Autodesk Fusion 360 part; units mm, degrees
note: some values were not read from the file. Set by a fixed rule: which face or edge a step refers to.
(part 2 of 3)
sketch "Skizze9" plane through (0, 0, 0) normal (0, 0, -1) x (1, 0, 0)
  circle A0 centre (287.3074, 352.379) radius 12
  line L0 (376.8151, 422.379) -> (364.2997, 422.379)
  arc A1 (343.5151, 422.379) -> (364.2997, 422.379) centre (353.9074, 428.379) ccw
  line L1 (343.5151, 422.379) -> (330.9997, 422.379)
  arc A2 (310.2151, 422.379) -> (330.9997, 422.379) centre (320.6074, 428.379) ccw
  line L2 (310.2151, 422.379) -> (297.6997, 422.379)
  arc A3 (276.9151, 422.379) -> (297.6997, 422.379) centre (287.3074, 428.379) ccw
  line L3 (276.9151, 422.379) -> (264.3997, 422.379)
  arc A4 (243.6151, 422.379) -> (264.3997, 422.379) centre (254.0074, 428.379) ccw
  line L4 (243.6151, 422.379) -> (231.0997, 422.379)
  arc A5 (210.3151, 422.379) -> (231.0997, 422.379) centre (220.7074, 428.379) ccw
  line L5 (210.3151, 422.379) -> (197.7997, 422.379)
  arc A6 (177.0151, 422.379) -> (197.7997, 422.379) centre (187.4074, 428.379) ccw
  line L6 (177.0151, 422.379) -> (164.4997, 422.379)
  arc A7 (143.7151, 422.379) -> (164.4997, 422.379) centre (154.1074, 428.379) ccw
  line L7 (143.7151, 422.379) -> (131.1997, 422.379)
  arc A8 (110.4151, 422.379) -> (131.1997, 422.379) centre (120.8074, 428.379) ccw
  line L8 (110.4151, 422.379) -> (97.8997, 422.379)
  arc A9 (77.1151, 422.379) -> (97.8997, 422.379) centre (87.5074, 428.379) ccw
  line L9 (77.1151, 422.379) -> (60.1074, 422.379)
  line L10 (60.1074, 422.379) -> (60.1074, 64.779)
  line L11 (60.1074, 64.779) -> (447.9074, 64.779)
  line L12 (447.9074, 64.779) -> (447.9074, 422.379)
  line L13 (447.9074, 422.379) -> (430.8997, 422.379)
  arc A10 (410.1151, 422.379) -> (430.8997, 422.379) centre (420.5074, 428.379) ccw
  line L14 (410.1151, 422.379) -> (397.5997, 422.379)
  arc A11 (376.8151, 422.379) -> (397.5997, 422.379) centre (387.2074, 428.379) ccw
  circle A12 centre (420.5074, 390.379) radius 12
  circle A13 centre (387.2074, 390.379) radius 12
  circle A14 centre (353.9074, 390.379) radius 12
  circle A15 centre (320.6074, 390.379) radius 12
  circle A16 centre (287.3074, 390.379) radius 12
  circle A17 centre (254.0074, 390.379) radius 12
  circle A18 centre (220.7074, 390.379) radius 12
  circle A19 centre (187.4074, 390.379) radius 12
  circle A20 centre (154.1074, 390.379) radius 12
  circle A21 centre (120.8074, 390.379) radius 12
  circle A22 centre (87.5074, 390.379) radius 12
  circle A23 centre (420.5074, 352.379) radius 12
  circle A24 centre (387.2074, 352.379) radius 12
  circle A25 centre (353.9074, 352.379) radius 12
  circle A26 centre (320.6074, 352.379) radius 12
  circle A27 centre (420.5074, 124.379) radius 12
  circle A28 centre (87.5074, 162.379) radius 12
  circle A29 centre (120.8074, 162.379) radius 12
  circle A30 centre (154.1074, 162.379) radius 12
  circle A31 centre (187.4074, 162.379) radius 12
  circle A32 centre (220.7074, 162.379) radius 12
  circle A33 centre (254.0074, 162.379) radius 12
  circle A34 centre (287.3074, 162.379) radius 12
  circle A35 centre (320.6074, 162.379) radius 12
  circle A36 centre (353.9074, 162.379) radius 12
  circle A37 centre (387.2074, 162.379) radius 12
  circle A38 centre (420.5074, 162.379) radius 12
  circle A39 centre (87.5074, 200.379) radius 12
  circle A40 centre (120.8074, 200.379) radius 12
  circle A41 centre (154.1074, 200.379) radius 12
  circle A42 centre (187.4074, 200.379) radius 12
  circle A43 centre (220.7074, 200.379) radius 12
  circle A44 centre (254.0074, 200.379) radius 12
  circle A45 centre (287.3074, 200.379) radius 12
  circle A46 centre (320.6074, 200.379) radius 12
  circle A47 centre (353.9074, 200.379) radius 12
  circle A48 centre (387.2074, 200.379) radius 12
  circle A49 centre (420.5074, 200.379) radius 12
  circle A50 centre (87.5074, 238.379) radius 12
  circle A51 centre (120.8074, 238.379) radius 12
  circle A52 centre (154.1074, 238.379) radius 12
  circle A53 centre (187.4074, 238.379) radius 12
  circle A54 centre (220.7074, 238.379) radius 12
  circle A55 centre (254.0074, 238.379) radius 12
  circle A56 centre (287.3074, 238.379) radius 12
  circle A57 centre (320.6074, 238.379) radius 12
  circle A58 centre (353.9074, 238.379) radius 12
  circle A59 centre (254.0074, 352.379) radius 12
  circle A60 centre (220.7074, 352.379) radius 12
  circle A61 centre (187.4074, 352.379) radius 12
  circle A62 centre (154.1074, 352.379) radius 12
  circle A63 centre (120.8074, 352.379) radius 12
  circle A64 centre (87.5074, 352.379) radius 12
  circle A65 centre (420.5074, 314.379) radius 12
  circle A66 centre (387.2074, 314.379) radius 12
  circle A67 centre (353.9074, 314.379) radius 12
  circle A68 centre (320.6074, 314.379) radius 12
  circle A69 centre (287.3074, 314.379) radius 12
  circle A70 centre (254.0074, 314.379) radius 12
  circle A71 centre (220.7074, 314.379) radius 12
  circle A72 centre (187.4074, 314.379) radius 12
  circle A73 centre (154.1074, 314.379) radius 12
  circle A74 centre (120.8074, 314.379) radius 12
  circle A75 centre (87.5074, 314.379) radius 12
  circle A76 centre (420.5074, 276.379) radius 12
  circle A77 centre (387.2074, 276.379) radius 12
  circle A78 centre (353.9074, 276.379) radius 12
  circle A79 centre (320.6074, 276.379) radius 12
  circle A80 centre (287.3074, 276.379) radius 12
  circle A81 centre (254.0074, 276.379) radius 12
  circle A82 centre (220.7074, 276.379) radius 12
  circle A83 centre (187.4074, 276.379) radius 12
  circle A84 centre (154.1074, 276.379) radius 12
  circle A85 centre (120.8074, 276.379) radius 12
  circle A86 centre (87.5074, 276.379) radius 12
  circle A87 centre (420.5074, 238.379) radius 12
  circle A88 centre (387.2074, 238.379) radius 12
  circle A89 centre (87.5074, 86.379) radius 12
  circle A90 centre (120.8074, 86.379) radius 12
  circle A91 centre (154.1074, 86.379) radius 12
  circle A92 centre (187.4074, 86.379) radius 12
  circle A93 centre (220.7074, 86.379) radius 12
  circle A94 centre (254.0074, 86.379) radius 12
  circle A95 centre (287.3074, 86.379) radius 12
  circle A96 centre (320.6074, 86.379) radius 12
  circle A97 centre (353.9074, 86.379) radius 12
  circle A98 centre (387.2074, 86.379) radius 12
  circle A99 centre (420.5074, 86.379) radius 12
  circle A100 centre (87.5074, 124.379) radius 12
  circle A101 centre (120.8074, 124.379) radius 12
  circle A102 centre (154.1074, 124.379) radius 12
  circle A103 centre (187.4074, 124.379) radius 12
  circle A104 centre (220.7074, 124.379) radius 12
  circle A105 centre (254.0074, 124.379) radius 12
  circle A106 centre (287.3074, 124.379) radius 12
  circle A107 centre (320.6074, 124.379) radius 12
  circle A108 centre (353.9074, 124.379) radius 12
  circle A109 centre (387.2074, 124.379) radius 12
  line L15 (60.1074, 396.379) -> (447.9074, 396.379)
  line L16 (447.9074, 396.379) -> (447.9074, 384.379)
  line L17 (447.9074, 384.379) -> (60.1074, 384.379)
  line L18 (60.1074, 384.379) -> (60.1074, 396.379)
  dimension "d208" = 6
  dimension "d209" = 6
  constraint horizontal L15
  constraint vertical L16
  constraint horizontal L17
  constraint vertical L18
  constraint collinear L10 L18
  constraint collinear L12 L16
  measures "d208" distance of A22.centre L15
  measures "d209" distance of A22.centre L17
extrude "Extrusion8" cut sketch "Skizze9" against normal blind 1 contours L12 A12 L15 L16 L17 | A12 A13 L15 L17 | L10 A22 L15 L17 L18 | A13 A14 L15 L17 | A21 A22 L15 L17 | A14 A15 L15 L17 | A20 A21 L15 L17 | A15 A16 L15 L17 | A19 A20 L15 L17 | A16 A17 L15 L17 | A18 A19 L15 L17 | A17 A18 L15 L17
extrude "Extrusion9" cut 1 faces at (441.9014, -440.073, 0) along direction (0, 0, 1) blind 10
extrude "Extrusion10" cut 1 faces at (441.4947, -412.7802, 0) along direction (0, 0, 1) blind 10
extrude "Extrusion11" cut 1 faces at (442.774, -216.5124, 0) along direction (0, 0, 1) blind 10
extrude "Extrusion12" cut 24 faces at (338.8297, -428.379, 1) (205.6297, -428.379, 1) (372.1297, -428.379, 1) (65.2519, -428.6779, 1) (305.5297, -428.379, 1) (272.2297, -428.379, 1) (238.9297, -428.379, 1) (105.7297, -428.379, 1) (172.3297, -428.379, 1) (139.0297, -428.379, 1) (405.4297, -428.379, 1) (442.774, -428.379, 1) (65.2519, -390.0801, 1) (105.7297, -390.379, 1) (139.0297, -390.379, 1) (172.3297, -390.379, 1) (205.6297, -390.379, 1) (238.9297, -390.379, 1) (272.2297, -390.379, 1) (305.5297, -390.379, 1) (338.8297, -390.379, 1) (372.1297, -390.379, 1) (405.4297, -390.379, 1) (442.774, -390.379, 1) along direction (0, 0, 1) blind 10
sketch "Skizze10" plane through (0, 0, 0) normal (0, 0, -1) x (1, 0, 0)
  line L0 (50.1074, 9.779) -> (50.1074, 49.779)
  line L1 (50.1074, 49.779) -> (10.1074, 49.779)
  line L2 (10.1074, 49.779) -> (10.1074, 464.979)
  line L3 (10.1074, 464.979) -> (50.1074, 464.979)
  line L4 (50.1074, 464.979) -> (50.1074, 504.979)
  line L5 (50.1074, 504.979) -> (457.9074, 504.979)
  line L6 (457.9074, 504.979) -> (457.9074, 464.979)
  line L7 (457.9074, 464.979) -> (497.9074, 464.979)
  line L8 (497.9074, 464.979) -> (497.9074, 49.779)
  line L9 (497.9074, 49.779) -> (457.9074, 49.779)
  line L10 (457.9074, 49.779) -> (457.9074, 9.779)
  line L11 (457.9074, 9.779) -> (50.1074, 9.779)
  circle A0 centre (479.9074, 23.779) radius 12
  circle A1 centre (28.1074, 23.779) radius 10.8095
  circle A2 centre (28.1074, 490.979) radius 12
  circle A3 centre (479.9074, 490.979) radius 12
  line L12 (507.9074, 514.979) -> (0.1074, 514.979)
  line L13 (0.1074, 514.979) -> (0.1074, -0.221)
  line L14 (0.1074, -0.221) -> (507.9074, -0.221)
  line L15 (507.9074, -0.221) -> (507.9074, 514.979)
  line L16 (457.9074, 496.979) -> (497.9074, 496.979)
  line L17 (497.9074, 496.979) -> (497.9074, 484.979)
  line L18 (497.9074, 484.979) -> (457.9074, 484.979)
  line L19 (457.9074, 484.979) -> (457.9074, 496.979)
  dimension "d220" = 6
  dimension "d221" = 6
  constraint horizontal L16
  constraint vertical L17
  constraint horizontal L18
  constraint vertical L19
  constraint coincident L6 L16.start
  constraint collinear L8 L17
  measures "d220" distance of A3.centre L16
  measures "d221" distance of A3.centre L18
extrude "Extrusion13" cut sketch "Skizze10" against normal blind 5 contours L6 A3 L16 L18 L19 | A3 L16 L17 L18
sketch "Skizze11" plane through (0, 0, 0) normal (0, 0, -1) x (1, 0, 0)
  line L0 (507.9074, 514.979) -> (0.1074, 514.979)
  line L1 (0.1074, 514.979) -> (0.1074, -0.221)
  line L2 (0.1074, -0.221) -> (507.9074, -0.221)
  line L3 (507.9074, -0.221) -> (507.9074, 514.979)
  circle A0 centre (28.1074, 490.979) radius 12
  circle A1 centre (28.1074, 23.779) radius 10.8095
  circle A2 centre (479.9074, 23.779) radius 12
  line L4 (469.5151, 484.979) -> (457.9074, 484.979)
  line L5 (457.9074, 484.979) -> (457.9074, 464.979)
  line L6 (457.9074, 464.979) -> (497.9074, 464.979)
  line L7 (497.9074, 464.979) -> (497.9074, 49.779)
  line L8 (497.9074, 49.779) -> (457.9074, 49.779)
  line L9 (457.9074, 49.779) -> (457.9074, 9.779)
  line L10 (457.9074, 9.779) -> (50.1074, 9.779)
  line L11 (50.1074, 9.779) -> (50.1074, 49.779)
  line L12 (50.1074, 49.779) -> (10.1074, 49.779)
  line L13 (10.1074, 49.779) -> (10.1074, 464.979)
  line L14 (10.1074, 464.979) -> (50.1074, 464.979)
  line L15 (50.1074, 464.979) -> (50.1074, 504.979)
  line L16 (50.1074, 504.979) -> (457.9074, 504.979)
  line L17 (457.9074, 504.979) -> (457.9074, 496.979)
  line L18 (457.9074, 496.979) -> (469.5151, 496.979)
  arc A3 (490.2997, 496.979) -> (469.5151, 496.979) centre (479.9074, 490.979) ccw
  line L19 (490.2997, 496.979) -> (497.9074, 496.979)
  line L20 (497.9074, 496.979) -> (497.9074, 484.979)
  line L21 (497.9074, 484.979) -> (490.2997, 484.979)
  arc A4 (469.5151, 484.979) -> (490.2997, 484.979) centre (479.9074, 490.979) ccw
  line L22 (10.1074, 496.979) -> (50.1074, 496.979)
  line L23 (50.1074, 496.979) -> (50.1074, 484.979)
  line L24 (50.1074, 484.979) -> (10.1074, 484.979)
  line L25 (10.1074, 484.979) -> (10.1074, 496.979)
  dimension "d224" = 6
  dimension "d225" = 6
  constraint horizontal L22
  constraint vertical L23
  constraint horizontal L24
  constraint vertical L25
  constraint collinear L15 L23
  constraint collinear L13 L25
  measures "d224" distance of A0.centre L22
  measures "d225" distance of A0.centre L24
extrude "Extrusion14" cut sketch "Skizze11" against normal blind 6 contours A0 L15 L22 L23 L24 | A0 L22 L24 L25
sketch "Skizze12" plane through (0, 0, 0) normal (0, 0, -1) x (1, 0, 0)
  line L0 (50.1074, 484.979) -> (38.4997, 484.979)
  arc A0 (17.7151, 484.979) -> (38.4997, 484.979) centre (28.1074, 490.979) ccw
  line L1 (17.7151, 484.979) -> (10.1074, 484.979)
  line L2 (10.1074, 484.979) -> (10.1074, 496.979)
  line L3 (10.1074, 496.979) -> (17.7151, 496.979)
  arc A1 (38.4997, 496.979) -> (17.7151, 496.979) centre (28.1074, 490.979) ccw
  line L4 (38.4997, 496.979) -> (50.1074, 496.979)
  line L5 (50.1074, 496.979) -> (50.1074, 504.979)
  line L6 (50.1074, 504.979) -> (457.9074, 504.979)
  line L7 (457.9074, 504.979) -> (457.9074, 496.979)
  line L8 (457.9074, 496.979) -> (469.5151, 496.979)
  arc A2 (490.2997, 496.979) -> (469.5151, 496.979) centre (479.9074, 490.979) ccw
  line L9 (490.2997, 496.979) -> (497.9074, 496.979)
  line L10 (497.9074, 496.979) -> (497.9074, 484.979)
  line L11 (497.9074, 484.979) -> (490.2997, 484.979)
  arc A3 (469.5151, 484.979) -> (490.2997, 484.979) centre (479.9074, 490.979) ccw
  line L12 (469.5151, 484.979) -> (457.9074, 484.979)
  line L13 (457.9074, 484.979) -> (457.9074, 464.979)
  line L14 (457.9074, 464.979) -> (497.9074, 464.979)
  line L15 (497.9074, 464.979) -> (497.9074, 49.779)
  line L16 (497.9074, 49.779) -> (457.9074, 49.779)
  line L17 (457.9074, 49.779) -> (457.9074, 9.779)
  line L18 (457.9074, 9.779) -> (50.1074, 9.779)
  line L19 (50.1074, 9.779) -> (50.1074, 49.779)
  line L20 (50.1074, 49.779) -> (10.1074, 49.779)
  line L21 (10.1074, 49.779) -> (10.1074, 464.979)
  line L22 (10.1074, 464.979) -> (50.1074, 464.979)
  line L23 (50.1074, 464.979) -> (50.1074, 484.979)
  line L24 (507.9074, 514.979) -> (0.1074, 514.979)
  line L25 (0.1074, 514.979) -> (0.1074, -0.221)
  line L26 (0.1074, -0.221) -> (507.9074, -0.221)
  line L27 (507.9074, -0.221) -> (507.9074, 514.979)
  circle A4 centre (28.1074, 23.779) radius 10.8095
  circle A5 centre (479.9074, 23.779) radius 12
  line L28 (10.1074, 29.779) -> (50.1074, 29.779)
  line L29 (50.1074, 29.779) -> (50.1074, 17.779)
  line L30 (50.1074, 17.779) -> (10.1074, 17.779)
  line L31 (10.1074, 17.779) -> (10.1074, 29.779)
  dimension "d228" = 6
  dimension "d229" = 6
  constraint horizontal L28
  constraint vertical L29
  constraint horizontal L30
  constraint vertical L31
  constraint collinear L19 L29
  constraint collinear L21 L31
  measures "d228" distance of A4.centre L28
  measures "d229" distance of A4.centre L30
extrude "Extrusion15" cut sketch "Skizze12" against normal blind 6 contours L19 A4 L28 L29 L30 | A4 L28 L30 L31
sketch "Skizze13" plane through (0, 0, 0) normal (0, 0, -1) x (1, 0, 0)
  line L0 (50.1074, 17.779) -> (37.0987, 17.779)
  arc A0 (19.116, 17.779) -> (37.0987, 17.779) centre (28.1074, 23.779) ccw
  line L1 (19.116, 17.779) -> (10.1074, 17.779)
  line L2 (10.1074, 17.779) -> (10.1074, 29.779)
  line L3 (10.1074, 29.779) -> (19.116, 29.779)
  arc A1 (37.0987, 29.779) -> (19.116, 29.779) centre (28.1074, 23.779) ccw
  line L4 (37.0987, 29.779) -> (50.1074, 29.779)
  line L5 (50.1074, 29.779) -> (50.1074, 49.779)
  line L6 (50.1074, 49.779) -> (10.1074, 49.779)
  line L7 (10.1074, 49.779) -> (10.1074, 464.979)
  line L8 (10.1074, 464.979) -> (50.1074, 464.979)
  line L9 (50.1074, 464.979) -> (50.1074, 484.979)
  line L10 (50.1074, 484.979) -> (38.4997, 484.979)
  arc A2 (17.7151, 484.979) -> (38.4997, 484.979) centre (28.1074, 490.979) ccw
  line L11 (17.7151, 484.979) -> (10.1074, 484.979)
  line L12 (10.1074, 484.979) -> (10.1074, 496.979)
  line L13 (10.1074, 496.979) -> (17.7151, 496.979)
  arc A3 (38.4997, 496.979) -> (17.7151, 496.979) centre (28.1074, 490.979) ccw
  line L14 (38.4997, 496.979) -> (50.1074, 496.979)
  line L15 (50.1074, 496.979) -> (50.1074, 504.979)
  line L16 (50.1074, 504.979) -> (457.9074, 504.979)
  line L17 (457.9074, 504.979) -> (457.9074, 496.979)
  line L18 (457.9074, 496.979) -> (469.5151, 496.979)
  arc A4 (490.2997, 496.979) -> (469.5151, 496.979) centre (479.9074, 490.979) ccw
  line L19 (490.2997, 496.979) -> (497.9074, 496.979)
  line L20 (497.9074, 496.979) -> (497.9074, 484.979)
  line L21 (497.9074, 484.979) -> (490.2997, 484.979)
  arc A5 (469.5151, 484.979) -> (490.2997, 484.979) centre (479.9074, 490.979) ccw
  line L22 (469.5151, 484.979) -> (457.9074, 484.979)
  line L23 (457.9074, 484.979) -> (457.9074, 464.979)
  line L24 (457.9074, 464.979) -> (497.9074, 464.979)
  line L25 (497.9074, 464.979) -> (497.9074, 49.779)
  line L26 (497.9074, 49.779) -> (457.9074, 49.779)
  line L27 (457.9074, 49.779) -> (457.9074, 9.779)
  line L28 (457.9074, 9.779) -> (50.1074, 9.779)
  line L29 (50.1074, 9.779) -> (50.1074, 17.779)
  line L30 (507.9074, 514.979) -> (0.1074, 514.979)
  line L31 (0.1074, 514.979) -> (0.1074, -0.221)
  line L32 (0.1074, -0.221) -> (507.9074, -0.221)
  line L33 (507.9074, -0.221) -> (507.9074, 514.979)
  circle A6 centre (479.9074, 23.779) radius 12
  line L34 (457.9074, 29.779) -> (497.9074, 29.779)
  line L35 (497.9074, 29.779) -> (497.9074, 17.779)
  line L36 (497.9074, 17.779) -> (457.9074, 17.779)
  line L37 (457.9074, 17.779) -> (457.9074, 29.779)
  dimension "d232" = 6
  dimension "d233" = 6
  constraint horizontal L34
  constraint vertical L35
  constraint horizontal L36
  constraint vertical L37
  constraint collinear L25 L35
  constraint collinear L27 L37
  measures "d232" distance of A6.centre L34
  measures "d233" distance of A6.centre L36
extrude "Extrusion16" cut sketch "Skizze13" against normal blind 6 contours L27 A6 L34 L36 L37 | A6 L34 L35 L36
sketch "Skizze14" plane through (0, 0, 10) normal (0, 0, -1) x (1, 0, 0)
  circle A0 centre (387.2074, 124.379) radius 12
  circle A1 centre (353.9074, 124.379) radius 12
  circle A2 centre (320.6074, 124.379) radius 12
  circle A3 centre (287.3074, 124.379) radius 12
  circle A4 centre (254.0074, 124.379) radius 12
  circle A5 centre (220.7074, 124.379) radius 12
  circle A6 centre (187.4074, 124.379) radius 12
  circle A7 centre (154.1074, 124.379) radius 12
  circle A8 centre (120.8074, 124.379) radius 12
  circle A9 centre (87.5074, 124.379) radius 12
  circle A10 centre (420.5074, 86.379) radius 12
  circle A11 centre (387.2074, 86.379) radius 12
  circle A12 centre (353.9074, 86.379) radius 12
  circle A13 centre (320.6074, 86.379) radius 12
  circle A14 centre (287.3074, 86.379) radius 12
  circle A15 centre (254.0074, 86.379) radius 12
  circle A16 centre (220.7074, 86.379) radius 12
  circle A17 centre (187.4074, 86.379) radius 12
  circle A18 centre (154.1074, 86.379) radius 12
  circle A19 centre (120.8074, 86.379) radius 12
  circle A20 centre (87.5074, 86.379) radius 12
  circle A21 centre (387.2074, 238.379) radius 12
  circle A22 centre (420.5074, 238.379) radius 12
  circle A23 centre (87.5074, 276.379) radius 12
  circle A24 centre (120.8074, 276.379) radius 12
  circle A25 centre (154.1074, 276.379) radius 12
  circle A26 centre (187.4074, 276.379) radius 12
  circle A27 centre (220.7074, 276.379) radius 12
  circle A28 centre (254.0074, 276.379) radius 12
  circle A29 centre (287.3074, 276.379) radius 12
  circle A30 centre (320.6074, 276.379) radius 12
  circle A31 centre (353.9074, 276.379) radius 12
  circle A32 centre (387.2074, 276.379) radius 12
  circle A33 centre (420.5074, 276.379) radius 12
  circle A34 centre (87.5074, 314.379) radius 12
  circle A35 centre (120.8074, 314.379) radius 12
  circle A36 centre (154.1074, 314.379) radius 12
  circle A37 centre (187.4074, 314.379) radius 12
  circle A38 centre (220.7074, 314.379) radius 12
  circle A39 centre (254.0074, 314.379) radius 12
  circle A40 centre (287.3074, 314.379) radius 12
  circle A41 centre (320.6074, 314.379) radius 12
  circle A42 centre (353.9074, 314.379) radius 12
  circle A43 centre (387.2074, 314.379) radius 12
  circle A44 centre (420.5074, 314.379) radius 12
  circle A45 centre (87.5074, 352.379) radius 12
  circle A46 centre (120.8074, 352.379) radius 12
  circle A47 centre (154.1074, 352.379) radius 12
  circle A48 centre (187.4074, 352.379) radius 12
  circle A49 centre (220.7074, 352.379) radius 12
  circle A50 centre (254.0074, 352.379) radius 12
  circle A51 centre (353.9074, 238.379) radius 12
  circle A52 centre (320.6074, 238.379) radius 12
  circle A53 centre (287.3074, 238.379) radius 12
  circle A54 centre (254.0074, 238.379) radius 12
  circle A55 centre (220.7074, 238.379) radius 12
  circle A56 centre (187.4074, 238.379) radius 12
  circle A57 centre (154.1074, 238.379) radius 12
  circle A58 centre (120.8074, 238.379) radius 12
  circle A59 centre (87.5074, 238.379) radius 12
  circle A60 centre (420.5074, 200.379) radius 12
  circle A61 centre (387.2074, 200.379) radius 12
  circle A62 centre (353.9074, 200.379) radius 12
  circle A63 centre (320.6074, 200.379) radius 12
  circle A64 centre (287.3074, 200.379) radius 12
  circle A65 centre (254.0074, 200.379) radius 12
  circle A66 centre (220.7074, 200.379) radius 12
  circle A67 centre (187.4074, 200.379) radius 12
  circle A68 centre (154.1074, 200.379) radius 12
  circle A69 centre (120.8074, 200.379) radius 12
  circle A70 centre (87.5074, 200.379) radius 12
  circle A71 centre (420.5074, 162.379) radius 12
  circle A72 centre (387.2074, 162.379) radius 12
  circle A73 centre (353.9074, 162.379) radius 12
  circle A74 centre (320.6074, 162.379) radius 12
  circle A75 centre (287.3074, 162.379) radius 12
  circle A76 centre (254.0074, 162.379) radius 12
  circle A77 centre (220.7074, 162.379) radius 12
  circle A78 centre (187.4074, 162.379) radius 12
  circle A79 centre (154.1074, 162.379) radius 12
  circle A80 centre (120.8074, 162.379) radius 12
  circle A81 centre (87.5074, 162.379) radius 12
  circle A82 centre (420.5074, 124.379) radius 12
  circle A83 centre (320.6074, 352.379) radius 12
  circle A84 centre (353.9074, 352.379) radius 12
  circle A85 centre (387.2074, 352.379) radius 12
  circle A86 centre (420.5074, 352.379) radius 12
  line L0 (376.8151, 384.379) -> (364.2997, 384.379)
  arc A87 (343.5151, 384.379) -> (364.2997, 384.379) centre (353.9074, 390.379) ccw
  line L1 (343.5151, 384.379) -> (330.9997, 384.379)
  arc A88 (310.2151, 384.379) -> (330.9997, 384.379) centre (320.6074, 390.379) ccw
  line L2 (310.2151, 384.379) -> (297.6997, 384.379)
  arc A89 (276.9151, 384.379) -> (297.6997, 384.379) centre (287.3074, 390.379) ccw
  line L3 (276.9151, 384.379) -> (264.3997, 384.379)
  arc A90 (243.6151, 384.379) -> (264.3997, 384.379) centre (254.0074, 390.379) ccw
  line L4 (243.6151, 384.379) -> (231.0997, 384.379)
  arc A91 (210.3151, 384.379) -> (231.0997, 384.379) centre (220.7074, 390.379) ccw
  line L5 (210.3151, 384.379) -> (197.7997, 384.379)
  arc A92 (177.0151, 384.379) -> (197.7997, 384.379) centre (187.4074, 390.379) ccw
  line L6 (177.0151, 384.379) -> (164.4997, 384.379)
  arc A93 (143.7151, 384.379) -> (164.4997, 384.379) centre (154.1074, 390.379) ccw
  line L7 (143.7151, 384.379) -> (131.1997, 384.379)
  arc A94 (110.4151, 384.379) -> (131.1997, 384.379) centre (120.8074, 390.379) ccw
  line L8 (110.4151, 384.379) -> (97.8997, 384.379)
  arc A95 (77.1151, 384.379) -> (97.8997, 384.379) centre (87.5074, 390.379) ccw
  line L9 (77.1151, 384.379) -> (60.1074, 384.379)
  line L10 (60.1074, 384.379) -> (60.1074, 64.779)
  line L11 (60.1074, 64.779) -> (447.9074, 64.779)
  line L12 (447.9074, 64.779) -> (447.9074, 384.379)
  line L13 (447.9074, 384.379) -> (430.8997, 384.379)
  arc A96 (410.1151, 384.379) -> (430.8997, 384.379) centre (420.5074, 390.379) ccw
  line L14 (410.1151, 384.379) -> (397.5997, 384.379)
  arc A97 (376.8151, 384.379) -> (397.5997, 384.379) centre (387.2074, 390.379) ccw
  circle A98 centre (287.3074, 352.379) radius 12
  line L15 (60.1074, 358.379) -> (447.9074, 358.379)
  line L16 (447.9074, 358.379) -> (447.9074, 346.379)
  line L17 (447.9074, 346.379) -> (60.1074, 346.379)
  line L18 (60.1074, 346.379) -> (60.1074, 358.379)
  dimension "d236" = 6
  dimension "d237" = 6
  constraint horizontal L15
  constraint vertical L16
  constraint horizontal L17
  constraint vertical L18
  constraint collinear L10 L18
  constraint collinear L12 L16
  measures "d236" distance of A45.centre L15
  measures "d237" distance of A45.centre L17
extrude "Extrusion17" cut sketch "Skizze14" against normal blind 1 contours A45 A46 L15 L17 | A45 L10 L15 L17 L18 | A46 A47 L15 L17 | A47 A48 L15 L17 | A86 L12 L15 L16 L17 | A48 A49 L15 L17 | A85 A86 L15 L17 | A49 A50 L15 L17 | A84 A85 L15 L17 | A50 A98 L15 L17 | A83 A84 L15 L17 | A83 A98 L15 L17
sketch "Skizze15" plane through (0, 0, 10) normal (0, 0, -1) x (1, 0, 0)
  line L0 (376.8151, 346.379) -> (364.2997, 346.379)
  arc A0 (343.5151, 346.379) -> (364.2997, 346.379) centre (353.9074, 352.379) ccw
  line L1 (343.5151, 346.379) -> (330.9997, 346.379)
  arc A1 (310.2151, 346.379) -> (330.9997, 346.379) centre (320.6074, 352.379) ccw
  line L2 (310.2151, 346.379) -> (297.6997, 346.379)
  arc A2 (276.9151, 346.379) -> (297.6997, 346.379) centre (287.3074, 352.379) ccw
  line L3 (276.9151, 346.379) -> (264.3997, 346.379)
  arc A3 (243.6151, 346.379) -> (264.3997, 346.379) centre (254.0074, 352.379) ccw
  line L4 (243.6151, 346.379) -> (231.0997, 346.379)
  arc A4 (210.3151, 346.379) -> (231.0997, 346.379) centre (220.7074, 352.379) ccw
  line L5 (210.3151, 346.379) -> (197.7997, 346.379)
  arc A5 (177.0151, 346.379) -> (197.7997, 346.379) centre (187.4074, 352.379) ccw
  line L6 (177.0151, 346.379) -> (164.4997, 346.379)
  arc A6 (143.7151, 346.379) -> (164.4997, 346.379) centre (154.1074, 352.379) ccw
  line L7 (143.7151, 346.379) -> (131.1997, 346.379)
  arc A7 (110.4151, 346.379) -> (131.1997, 346.379) centre (120.8074, 352.379) ccw
  line L8 (110.4151, 346.379) -> (97.8997, 346.379)
  arc A8 (77.1151, 346.379) -> (97.8997, 346.379) centre (87.5074, 352.379) ccw
  line L9 (77.1151, 346.379) -> (60.1074, 346.379)
  line L10 (60.1074, 346.379) -> (60.1074, 64.779)
  line L11 (60.1074, 64.779) -> (447.9074, 64.779)
  line L12 (447.9074, 64.779) -> (447.9074, 346.379)
  line L13 (447.9074, 346.379) -> (430.8997, 346.379)
  arc A9 (410.1151, 346.379) -> (430.8997, 346.379) centre (420.5074, 352.379) ccw
  line L14 (410.1151, 346.379) -> (397.5997, 346.379)
  arc A10 (376.8151, 346.379) -> (397.5997, 346.379) centre (387.2074, 352.379) ccw
  circle A11 centre (420.5074, 124.379) radius 12
  circle A12 centre (87.5074, 162.379) radius 12
  circle A13 centre (120.8074, 162.379) radius 12
  circle A14 centre (154.1074, 162.379) radius 12
  circle A15 centre (187.4074, 162.379) radius 12
  circle A16 centre (220.7074, 162.379) radius 12
  circle A17 centre (254.0074, 162.379) radius 12
  circle A18 centre (287.3074, 162.379) radius 12
  circle A19 centre (320.6074, 162.379) radius 12
  circle A20 centre (353.9074, 162.379) radius 12
  circle A21 centre (387.2074, 162.379) radius 12
  circle A22 centre (420.5074, 162.379) radius 12
  circle A23 centre (87.5074, 200.379) radius 12
  circle A24 centre (120.8074, 200.379) radius 12
  circle A25 centre (154.1074, 200.379) radius 12
  circle A26 centre (187.4074, 200.379) radius 12
  circle A27 centre (220.7074, 200.379) radius 12
  circle A28 centre (254.0074, 200.379) radius 12
  circle A29 centre (287.3074, 200.379) radius 12
  circle A30 centre (320.6074, 200.379) radius 12
  circle A31 centre (353.9074, 200.379) radius 12
  circle A32 centre (387.2074, 200.379) radius 12
  circle A33 centre (420.5074, 200.379) radius 12
  circle A34 centre (87.5074, 238.379) radius 12
  circle A35 centre (120.8074, 238.379) radius 12
  circle A36 centre (154.1074, 238.379) radius 12
  circle A37 centre (187.4074, 238.379) radius 12
  circle A38 centre (220.7074, 238.379) radius 12
  circle A39 centre (254.0074, 238.379) radius 12
  circle A40 centre (287.3074, 238.379) radius 12
  circle A41 centre (320.6074, 238.379) radius 12
  circle A42 centre (353.9074, 238.379) radius 12
  circle A43 centre (420.5074, 314.379) radius 12
  circle A44 centre (387.2074, 314.379) radius 12
  circle A45 centre (353.9074, 314.379) radius 12
  circle A46 centre (320.6074, 314.379) radius 12
  circle A47 centre (287.3074, 314.379) radius 12
  circle A48 centre (254.0074, 314.379) radius 12
  circle A49 centre (220.7074, 314.379) radius 12
  circle A50 centre (187.4074, 314.379) radius 12
  circle A51 centre (154.1074, 314.379) radius 12
  circle A52 centre (120.8074, 314.379) radius 12
  circle A53 centre (87.5074, 314.379) radius 12
  circle A54 centre (420.5074, 276.379) radius 12
  circle A55 centre (387.2074, 276.379) radius 12
  circle A56 centre (353.9074, 276.379) radius 12
  circle A57 centre (320.6074, 276.379) radius 12
  circle A58 centre (287.3074, 276.379) radius 12
  circle A59 centre (254.0074, 276.379) radius 12
  circle A60 centre (220.7074, 276.379) radius 12
  circle A61 centre (187.4074, 276.379) radius 12
  circle A62 centre (154.1074, 276.379) radius 12
  circle A63 centre (120.8074, 276.379) radius 12
  circle A64 centre (87.5074, 276.379) radius 12
  circle A65 centre (420.5074, 238.379) radius 12
  circle A66 centre (387.2074, 238.379) radius 12
  circle A67 centre (87.5074, 86.379) radius 12
  circle A68 centre (120.8074, 86.379) radius 12
  circle A69 centre (154.1074, 86.379) radius 12
  circle A70 centre (187.4074, 86.379) radius 12
  circle A71 centre (220.7074, 86.379) radius 12
  circle A72 centre (254.0074, 86.379) radius 12
  circle A73 centre (287.3074, 86.379) radius 12
  circle A74 centre (320.6074, 86.379) radius 12
  circle A75 centre (353.9074, 86.379) radius 12
  circle A76 centre (387.2074, 86.379) radius 12
  circle A77 centre (420.5074, 86.379) radius 12
  circle A78 centre (87.5074, 124.379) radius 12
  circle A79 centre (120.8074, 124.379) radius 12
  circle A80 centre (154.1074, 124.379) radius 12
  circle A81 centre (187.4074, 124.379) radius 12
  circle A82 centre (220.7074, 124.379) radius 12
  circle A83 centre (254.0074, 124.379) radius 12
  circle A84 centre (287.3074, 124.379) radius 12
  circle A85 centre (320.6074, 124.379) radius 12
  circle A86 centre (353.9074, 124.379) radius 12
  circle A87 centre (387.2074, 124.379) radius 12
  line L15 (60.1074, 320.379) -> (447.9074, 320.379)
  line L16 (447.9074, 320.379) -> (447.9074, 308.379)
  line L17 (447.9074, 308.379) -> (60.1074, 308.379)
  line L18 (60.1074, 308.379) -> (60.1074, 320.379)
  dimension "d240" = 6
  dimension "d241" = 6
  constraint horizontal L15
  constraint vertical L16
  constraint horizontal L17
  constraint vertical L18
  constraint collinear L10 L18
  constraint collinear L12 L16
  measures "d240" distance of A53.centre L17
  measures "d241" distance of A53.centre L15
extrude "Extrusion18" cut sketch "Skizze15" against normal blind 1 contours L12 A43 L15 L16 L17 | A43 A44 L15 L17 | L10 A53 L15 L17 L18 | A44 A45 L15 L17 | A52 A53 L15 L17 | A45 A46 L15 L17 | A51 A52 L15 L17 | A46 A47 L15 L17 | A50 A51 L15 L17 | A47 A48 L15 L17 | A49 A50 L15 L17 | A48 A49 L15 L17
sketch "Skizze16" plane through (0, 0, 10) normal (0, 0, -1) x (1, 0, 0)
  circle A0 centre (387.2074, 124.379) radius 12
  circle A1 centre (353.9074, 124.379) radius 12
  circle A2 centre (320.6074, 124.379) radius 12
  circle A3 centre (287.3074, 124.379) radius 12
  circle A4 centre (254.0074, 124.379) radius 12
  circle A5 centre (220.7074, 124.379) radius 12
  circle A6 centre (187.4074, 124.379) radius 12
  circle A7 centre (154.1074, 124.379) radius 12
  circle A8 centre (120.8074, 124.379) radius 12
  circle A9 centre (87.5074, 124.379) radius 12
  circle A10 centre (420.5074, 86.379) radius 12
  circle A11 centre (387.2074, 86.379) radius 12
  circle A12 centre (353.9074, 86.379) radius 12
  circle A13 centre (320.6074, 86.379) radius 12
  circle A14 centre (287.3074, 86.379) radius 12
  circle A15 centre (254.0074, 86.379) radius 12
  circle A16 centre (220.7074, 86.379) radius 12
  circle A17 centre (187.4074, 86.379) radius 12
  circle A18 centre (154.1074, 86.379) radius 12
  circle A19 centre (120.8074, 86.379) radius 12
  circle A20 centre (87.5074, 86.379) radius 12
  circle A21 centre (387.2074, 238.379) radius 12
  circle A22 centre (420.5074, 238.379) radius 12
  circle A23 centre (87.5074, 276.379) radius 12
  circle A24 centre (120.8074, 276.379) radius 12
  circle A25 centre (154.1074, 276.379) radius 12
  circle A26 centre (187.4074, 276.379) radius 12
  circle A27 centre (220.7074, 276.379) radius 12
  circle A28 centre (254.0074, 276.379) radius 12
  circle A29 centre (287.3074, 276.379) radius 12
  circle A30 centre (320.6074, 276.379) radius 12
  circle A31 centre (353.9074, 276.379) radius 12
  circle A32 centre (387.2074, 276.379) radius 12
  circle A33 centre (420.5074, 276.379) radius 12
  line L0 (376.8151, 308.379) -> (364.2997, 308.379)
  arc A34 (343.5151, 308.379) -> (364.2997, 308.379) centre (353.9074, 314.379) ccw
  line L1 (343.5151, 308.379) -> (330.9997, 308.379)
  arc A35 (310.2151, 308.379) -> (330.9997, 308.379) centre (320.6074, 314.379) ccw
  line L2 (310.2151, 308.379) -> (297.6997, 308.379)
  arc A36 (276.9151, 308.379) -> (297.6997, 308.379) centre (287.3074, 314.379) ccw
  line L3 (276.9151, 308.379) -> (264.3997, 308.379)
  arc A37 (243.6151, 308.379) -> (264.3997, 308.379) centre (254.0074, 314.379) ccw
  line L4 (243.6151, 308.379) -> (231.0997, 308.379)
  arc A38 (210.3151, 308.379) -> (231.0997, 308.379) centre (220.7074, 314.379) ccw
  line L5 (210.3151, 308.379) -> (197.7997, 308.379)
  arc A39 (177.0151, 308.379) -> (197.7997, 308.379) centre (187.4074, 314.379) ccw
  line L6 (177.0151, 308.379) -> (164.4997, 308.379)
  arc A40 (143.7151, 308.379) -> (164.4997, 308.379) centre (154.1074, 314.379) ccw
  line L7 (143.7151, 308.379) -> (131.1997, 308.379)
  arc A41 (110.4151, 308.379) -> (131.1997, 308.379) centre (120.8074, 314.379) ccw
  line L8 (110.4151, 308.379) -> (97.8997, 308.379)
  arc A42 (77.1151, 308.379) -> (97.8997, 308.379) centre (87.5074, 314.379) ccw
  line L9 (77.1151, 308.379) -> (60.1074, 308.379)
  line L10 (60.1074, 308.379) -> (60.1074, 64.779)
  line L11 (60.1074, 64.779) -> (447.9074, 64.779)
  line L12 (447.9074, 64.779) -> (447.9074, 308.379)
  line L13 (447.9074, 308.379) -> (430.8997, 308.379)
  arc A43 (410.1151, 308.379) -> (430.8997, 308.379) centre (420.5074, 314.379) ccw
  line L14 (410.1151, 308.379) -> (397.5997, 308.379)
  arc A44 (376.8151, 308.379) -> (397.5997, 308.379) centre (387.2074, 314.379) ccw
  circle A45 centre (353.9074, 238.379) radius 12
  circle A46 centre (320.6074, 238.379) radius 12
  circle A47 centre (287.3074, 238.379) radius 12
  circle A48 centre (254.0074, 238.379) radius 12
  circle A49 centre (220.7074, 238.379) radius 12
  circle A50 centre (187.4074, 238.379) radius 12
  circle A51 centre (154.1074, 238.379) radius 12
  circle A52 centre (120.8074, 238.379) radius 12
  circle A53 centre (87.5074, 238.379) radius 12
  circle A54 centre (420.5074, 200.379) radius 12
  circle A55 centre (387.2074, 200.379) radius 12
  circle A56 centre (353.9074, 200.379) radius 12
  circle A57 centre (320.6074, 200.379) radius 12
  circle A58 centre (287.3074, 200.379) radius 12
  circle A59 centre (254.0074, 200.379) radius 12
  circle A60 centre (220.7074, 200.379) radius 12
  circle A61 centre (187.4074, 200.379) radius 12
  circle A62 centre (154.1074, 200.379) radius 12
  circle A63 centre (120.8074, 200.379) radius 12
  circle A64 centre (87.5074, 200.379) radius 12
  circle A65 centre (420.5074, 162.379) radius 12
  circle A66 centre (387.2074, 162.379) radius 12
  circle A67 centre (353.9074, 162.379) radius 12
  circle A68 centre (320.6074, 162.379) radius 12
  circle A69 centre (287.3074, 162.379) radius 12
  circle A70 centre (254.0074, 162.379) radius 12
  circle A71 centre (220.7074, 162.379) radius 12
  circle A72 centre (187.4074, 162.379) radius 12
  circle A73 centre (154.1074, 162.379) radius 12
  circle A74 centre (120.8074, 162.379) radius 12
  circle A75 centre (87.5074, 162.379) radius 12
  circle A76 centre (420.5074, 124.379) radius 12
  line L15 (60.1074, 282.379) -> (447.9074, 282.379)
  line L16 (447.9074, 282.379) -> (447.9074, 270.379)
  line L17 (447.9074, 270.379) -> (60.1074, 270.379)
  line L18 (60.1074, 270.379) -> (60.1074, 282.379)
  dimension "d244" = 6
  dimension "d245" = 6
  constraint horizontal L15
  constraint vertical L16
  constraint horizontal L17
  constraint vertical L18
  constraint collinear L10 L18
  constraint collinear L12 L16
  measures "d244" distance of A23.centre L15
  measures "d245" distance of A23.centre L17
extrude "Extrusion19" cut sketch "Skizze16" against normal blind 1 contours A23 A24 L15 L17 | A23 L10 L15 L17 L18 | A24 A25 L15 L17 | A25 A26 L15 L17 | A33 L12 L15 L16 L17 | A26 A27 L15 L17 | A32 A33 L15 L17 | A27 A28 L15 L17 | A31 A32 L15 L17 | A28 A29 L15 L17 | A30 A31 L15 L17 | A29 A30 L15 L17
sketch "Skizze17" plane through (0, 0, 10) normal (0, 0, -1) x (1, 0, 0)
  circle A0 centre (420.5074, 124.379) radius 12
  circle A1 centre (87.5074, 162.379) radius 12
  circle A2 centre (120.8074, 162.379) radius 12
  circle A3 centre (154.1074, 162.379) radius 12
  circle A4 centre (187.4074, 162.379) radius 12
  circle A5 centre (220.7074, 162.379) radius 12
  circle A6 centre (254.0074, 162.379) radius 12
  circle A7 centre (287.3074, 162.379) radius 12
  circle A8 centre (320.6074, 162.379) radius 12
  circle A9 centre (353.9074, 162.379) radius 12
  circle A10 centre (387.2074, 162.379) radius 12
  circle A11 centre (420.5074, 162.379) radius 12
  circle A12 centre (87.5074, 200.379) radius 12
  circle A13 centre (120.8074, 200.379) radius 12
  circle A14 centre (154.1074, 200.379) radius 12
  circle A15 centre (187.4074, 200.379) radius 12
  circle A16 centre (220.7074, 200.379) radius 12
  circle A17 centre (254.0074, 200.379) radius 12
  circle A18 centre (287.3074, 200.379) radius 12
  circle A19 centre (320.6074, 200.379) radius 12
  circle A20 centre (353.9074, 200.379) radius 12
  circle A21 centre (387.2074, 200.379) radius 12
  circle A22 centre (420.5074, 200.379) radius 12
  circle A23 centre (87.5074, 238.379) radius 12
  circle A24 centre (120.8074, 238.379) radius 12
  circle A25 centre (154.1074, 238.379) radius 12
  circle A26 centre (187.4074, 238.379) radius 12
  circle A27 centre (220.7074, 238.379) radius 12
  circle A28 centre (254.0074, 238.379) radius 12
  circle A29 centre (287.3074, 238.379) radius 12
  circle A30 centre (320.6074, 238.379) radius 12
  circle A31 centre (353.9074, 238.379) radius 12
  line L0 (376.8151, 270.379) -> (364.2997, 270.379)
  arc A32 (343.5151, 270.379) -> (364.2997, 270.379) centre (353.9074, 276.379) ccw
  line L1 (343.5151, 270.379) -> (330.9997, 270.379)
  arc A33 (310.2151, 270.379) -> (330.9997, 270.379) centre (320.6074, 276.379) ccw
  line L2 (310.2151, 270.379) -> (297.6997, 270.379)
  arc A34 (276.9151, 270.379) -> (297.6997, 270.379) centre (287.3074, 276.379) ccw
  line L3 (276.9151, 270.379) -> (264.3997, 270.379)
  arc A35 (243.6151, 270.379) -> (264.3997, 270.379) centre (254.0074, 276.379) ccw
  line L4 (243.6151, 270.379) -> (231.0997, 270.379)
  arc A36 (210.3151, 270.379) -> (231.0997, 270.379) centre (220.7074, 276.379) ccw
  line L5 (210.3151, 270.379) -> (197.7997, 270.379)
  arc A37 (177.0151, 270.379) -> (197.7997, 270.379) centre (187.4074, 276.379) ccw
  line L6 (177.0151, 270.379) -> (164.4997, 270.379)
  arc A38 (143.7151, 270.379) -> (164.4997, 270.379) centre (154.1074, 276.379) ccw
  line L7 (143.7151, 270.379) -> (131.1997, 270.379)
  arc A39 (110.4151, 270.379) -> (131.1997, 270.379) centre (120.8074, 276.379) ccw
  line L8 (110.4151, 270.379) -> (97.8997, 270.379)
  arc A40 (77.1151, 270.379) -> (97.8997, 270.379) centre (87.5074, 276.379) ccw
  line L9 (77.1151, 270.379) -> (60.1074, 270.379)
  line L10 (60.1074, 270.379) -> (60.1074, 64.779)
  line L11 (60.1074, 64.779) -> (447.9074, 64.779)
  line L12 (447.9074, 64.779) -> (447.9074, 270.379)
  line L13 (447.9074, 270.379) -> (430.8997, 270.379)
  arc A41 (410.1151, 270.379) -> (430.8997, 270.379) centre (420.5074, 276.379) ccw
  line L14 (410.1151, 270.379) -> (397.5997, 270.379)
  arc A42 (376.8151, 270.379) -> (397.5997, 270.379) centre (387.2074, 276.379) ccw
  circle A43 centre (420.5074, 238.379) radius 12
  circle A44 centre (387.2074, 238.379) radius 12
  circle A45 centre (87.5074, 86.379) radius 12
  circle A46 centre (120.8074, 86.379) radius 12
  circle A47 centre (154.1074, 86.379) radius 12
  circle A48 centre (187.4074, 86.379) radius 12
  circle A49 centre (220.7074, 86.379) radius 12
  circle A50 centre (254.0074, 86.379) radius 12
  circle A51 centre (287.3074, 86.379) radius 12
  circle A52 centre (320.6074, 86.379) radius 12
  circle A53 centre (353.9074, 86.379) radius 12
  circle A54 centre (387.2074, 86.379) radius 12
  circle A55 centre (420.5074, 86.379) radius 12
  circle A56 centre (87.5074, 124.379) radius 12
  circle A57 centre (120.8074, 124.379) radius 12
  circle A58 centre (154.1074, 124.379) radius 12
  circle A59 centre (187.4074, 124.379) radius 12
  circle A60 centre (220.7074, 124.379) radius 12
  circle A61 centre (254.0074, 124.379) radius 12
  circle A62 centre (287.3074, 124.379) radius 12
  circle A63 centre (320.6074, 124.379) radius 12
  circle A64 centre (353.9074, 124.379) radius 12
  circle A65 centre (387.2074, 124.379) radius 12
  line L15 (60.1074, 244.379) -> (447.9074, 244.379)
  line L16 (447.9074, 244.379) -> (447.9074, 232.379)
  line L17 (447.9074, 232.379) -> (60.1074, 232.379)
  line L18 (60.1074, 232.379) -> (60.1074, 244.379)
  dimension "d248" = 6
  dimension "d249" = 6
  constraint horizontal L15
  constraint vertical L16
  constraint horizontal L17
  constraint vertical L18
  constraint collinear L10 L18
  constraint collinear L12 L16
  measures "d248" distance of A23.centre L15
  measures "d249" distance of A23.centre L17
extrude "Extrusion20" cut sketch "Skizze17" against normal blind 1 contours A23 A24 L15 L17 | A23 L10 L15 L17 L18 | A24 A25 L15 L17 | A25 A26 L15 L17 | L12 A43 L15 L16 L17 | A26 A27 L15 L17 | A43 A44 L15 L17 | A27 A28 L15 L17 | A31 A44 L15 L17 | A28 A29 L15 L17 | A30 A31 L15 L17 | A29 A30 L15 L17
sketch "Skizze18" plane through (0, 0, 10) normal (0, 0, -1) x (1, 0, 0)
  circle A0 centre (387.2074, 124.379) radius 12
  circle A1 centre (353.9074, 124.379) radius 12
  circle A2 centre (320.6074, 124.379) radius 12
  circle A3 centre (287.3074, 124.379) radius 12
  circle A4 centre (254.0074, 124.379) radius 12
  circle A5 centre (220.7074, 124.379) radius 12
  circle A6 centre (187.4074, 124.379) radius 12
  circle A7 centre (154.1074, 124.379) radius 12
  circle A8 centre (120.8074, 124.379) radius 12
  circle A9 centre (87.5074, 124.379) radius 12
  circle A10 centre (420.5074, 86.379) radius 12
  circle A11 centre (387.2074, 86.379) radius 12
  circle A12 centre (353.9074, 86.379) radius 12
  circle A13 centre (320.6074, 86.379) radius 12
  circle A14 centre (287.3074, 86.379) radius 12
  circle A15 centre (254.0074, 86.379) radius 12
  circle A16 centre (220.7074, 86.379) radius 12
  circle A17 centre (187.4074, 86.379) radius 12
  circle A18 centre (154.1074, 86.379) radius 12
  circle A19 centre (120.8074, 86.379) radius 12
  circle A20 centre (87.5074, 86.379) radius 12
  line L0 (376.8151, 232.379) -> (364.2997, 232.379)
  arc A21 (343.5151, 232.379) -> (364.2997, 232.379) centre (353.9074, 238.379) ccw
  line L1 (343.5151, 232.379) -> (330.9997, 232.379)
  arc A22 (310.2151, 232.379) -> (330.9997, 232.379) centre (320.6074, 238.379) ccw
  line L2 (310.2151, 232.379) -> (297.6997, 232.379)
  arc A23 (276.9151, 232.379) -> (297.6997, 232.379) centre (287.3074, 238.379) ccw
  line L3 (276.9151, 232.379) -> (264.3997, 232.379)
  arc A24 (243.6151, 232.379) -> (264.3997, 232.379) centre (254.0074, 238.379) ccw
  line L4 (243.6151, 232.379) -> (231.0997, 232.379)
  arc A25 (210.3151, 232.379) -> (231.0997, 232.379) centre (220.7074, 238.379) ccw
  line L5 (210.3151, 232.379) -> (197.7997, 232.379)
  arc A26 (177.0151, 232.379) -> (197.7997, 232.379) centre (187.4074, 238.379) ccw
  line L6 (177.0151, 232.379) -> (164.4997, 232.379)
  arc A27 (143.7151, 232.379) -> (164.4997, 232.379) centre (154.1074, 238.379) ccw
  line L7 (143.7151, 232.379) -> (131.1997, 232.379)
  arc A28 (110.4151, 232.379) -> (131.1997, 232.379) centre (120.8074, 238.379) ccw
  line L8 (110.4151, 232.379) -> (97.8997, 232.379)
  arc A29 (77.1151, 232.379) -> (97.8997, 232.379) centre (87.5074, 238.379) ccw
  line L9 (77.1151, 232.379) -> (60.1074, 232.379)
  line L10 (60.1074, 232.379) -> (60.1074, 64.779)
  line L11 (60.1074, 64.779) -> (447.9074, 64.779)
  line L12 (447.9074, 64.779) -> (447.9074, 232.379)
  line L13 (447.9074, 232.379) -> (430.8997, 232.379)
  arc A30 (410.1151, 232.379) -> (430.8997, 232.379) centre (420.5074, 238.379) ccw
  line L14 (410.1151, 232.379) -> (397.5997, 232.379)
  arc A31 (376.8151, 232.379) -> (397.5997, 232.379) centre (387.2074, 238.379) ccw
  circle A32 centre (420.5074, 200.379) radius 12
  circle A33 centre (387.2074, 200.379) radius 12
  circle A34 centre (353.9074, 200.379) radius 12
  circle A35 centre (320.6074, 200.379) radius 12
  circle A36 centre (287.3074, 200.379) radius 12
  circle A37 centre (254.0074, 200.379) radius 12
  circle A38 centre (220.7074, 200.379) radius 12
  circle A39 centre (187.4074, 200.379) radius 12
  circle A40 centre (154.1074, 200.379) radius 12
  circle A41 centre (120.8074, 200.379) radius 12
  circle A42 centre (87.5074, 200.379) radius 12
  circle A43 centre (420.5074, 162.379) radius 12
  circle A44 centre (387.2074, 162.379) radius 12
  circle A45 centre (353.9074, 162.379) radius 12
  circle A46 centre (320.6074, 162.379) radius 12
  circle A47 centre (287.3074, 162.379) radius 12
  circle A48 centre (254.0074, 162.379) radius 12
  circle A49 centre (220.7074, 162.379) radius 12
  circle A50 centre (187.4074, 162.379) radius 12
  circle A51 centre (154.1074, 162.379) radius 12
  circle A52 centre (120.8074, 162.379) radius 12
  circle A53 centre (87.5074, 162.379) radius 12
  circle A54 centre (420.5074, 124.379) radius 12
  line L15 (60.1074, 206.379) -> (447.9074, 206.379)
  line L16 (447.9074, 206.379) -> (447.9074, 194.379)
  line L17 (447.9074, 194.379) -> (60.1074, 194.379)
  line L18 (60.1074, 194.379) -> (60.1074, 206.379)
  dimension "d252" = 6
  dimension "d253" = 6
  constraint horizontal L15
  constraint vertical L16
  constraint horizontal L17
  constraint vertical L18
  constraint collinear L10 L18
  constraint collinear L12 L16
  measures "d252" distance of A42.centre L15
  measures "d253" distance of A42.centre L17
extrude "Extrusion21" cut sketch "Skizze18" against normal blind 1 contours L12 A32 L15 L16 L17 | A32 A33 L15 L17 | L10 A42 L15 L17 L18 | A33 A34 L15 L17 | A41 A42 L15 L17 | A34 A35 L15 L17 | A40 A41 L15 L17 | A35 A36 L15 L17 | A39 A40 L15 L17 | A36 A37 L15 L17 | A38 A39 L15 L17 | A37 A38 L15 L17